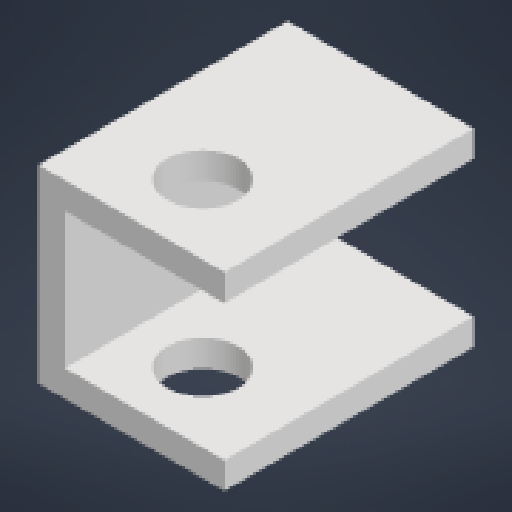
# Autodesk Inventor part: Part4
Saved by Autodesk Inventor 2026 (Build 300175000, 175)
## iProperties
Created: 2025-10-10
Part Number: Part4
Material: Generic
Document SubType Name: Modeling
Designer: kenny
Density: 1 g/cm^3
Appearance: Default
Author: kenny
Autodesk Inventor part; units mm, degrees
ref_plane "YZ Plane" through (0, 0, 0) normal (1, 0, 0) x (0, 1, 0)
ref_plane "XZ Plane" through (0, 0, 0) normal (0, 1, 0) x (-1, 0, 0)
ref_plane "XY Plane" through (0, 0, 0) normal (0, 0, 1) x (1, 0, 0)
sketch "Sketch1" plane through (0, 0, 0) normal (0, 0, 1) x (1, 0, 0)
  line L0 (-5.7, 0) -> (-5.7, -5.7)
  line L1 (-5.7, -5.7) -> (0, -5.7)
  line L2 (0, 5.7) -> (-5.7, 5.7)
  line L3 (-5.7, 5.7) -> (-5.7, 0)
  line L4 (0, 4.1) -> (-4.1, 4.1)
  line L5 (-4.1, 4.1) -> (-4.1, -4.1)
  line L6 (-4.1, -4.1) -> (0, -4.1)
  line L7 (3.9, -5.7) -> (0, -5.7)
  line L8 (3.9, 5.7) -> (0, 5.7)
  line L9 (3.9, 5.7) -> (5.5, 5.7)
  line L10 (3.9, -5.7) -> (5.5, -5.7)
  line L11 (5.5, 4.1) -> (0, 4.1)
  line L12 (5.5, -4.1) -> (0, -4.1)
  line L13 (0, 0) -> (4.1, 0)
  line L14 (4.1, 0) -> (5.7, 0)
  line L15 (5.7, 0) -> (5.7, 5.7)
  line L16 (5.7, 5.7) -> (5.5, 5.7)
  line L17 (5.5, 4.1) -> (5.7, 4.1)
  line L18 (5.7, 0) -> (5.7, -5.7)
  line L19 (5.7, -5.7) -> (5.5, -5.7)
  line L20 (5.5, -4.1) -> (5.7, -4.1)
  dimension "d22" = 4.1
  dimension "d23" = 1.6
  constraints: 42 end point, 8 perpendicular, 5 point on line, 3 horizontal, 2 collinear
  measures "d22" distance of L13.start L13.end
  measures "d23" distance of L13.end L14.end
extrude "Extrusion1" add sketch "Sketch1" against normal blind 15 contours L3 L2 L8 L9 L16 L15 L17 L11 L4 L5 L6 L12 L20 L18 L19 L10 L7 L1 L0
sketch "Sketch2" plane through (-5.7, 5.7, 0) normal (0, 1, 0) x (1, 0, 0)
  line L0 (5.7, 0) -> (5.7, 4.2)
  circle A0 centre (5.7, 4.2) radius 2.15
  dimension "d10" = 4.2
  dimension "d11" = 4.3
  constraints: 2 end point, 1 centre point, 1 coincident, 1 vertical
  measures "d10" distance of L0.start L0.end
  measures "d11" diameter of A0
extrude "Extrusion2" cut sketch "Sketch2" against normal blind 15
sketch "Sketch3" plane through (0, 0, 0) normal (0, 0, 1) x (1, 0, 0)
  point P0 (0, 0)
sketch "Sketch4" plane through (0, 0, 0) normal (0, 0, 1) x (1, 0, 0)
  point P0 (5.5, 5.7)
sketch "Sketch5" plane through (0, 0, 0) normal (0, 0, 1) x (1, 0, 0)
  line L0 (5.7, 4.1) -> (5.7, 0)
  line L1 (5.7, 0) -> (5.7, 24)
  line L2 (5.7, 0) -> (5.7, -24)
  line L3 (5.7, -25.6) -> (4.1, -25.6)
  line L4 (5.7, -5.7) -> (-5.7, -5.7) projected
  line L5 (4.1, -5.7) -> (4.1, -25.6)
  line L6 (5.7, 25.6) -> (4.1, 25.6)
  line L7 (4.1, 25.6) -> (4.1, 5.7)
  line L8 (5.7, 5.7) -> (-5.7, 5.7) projected
  line L9 (5.7, 25.6) -> (18.7, 25.6)
  line L10 (18.7, 25.6) -> (18.7, 24)
  line L11 (18.7, 24) -> (5.7, 24)
  line L12 (5.7, -25.6) -> (18.7, -25.6)
  line L13 (18.7, -25.6) -> (18.7, -24)
  line L14 (18.7, -24) -> (5.7, -24)
  line L15 (4.1, 5.7) -> (4.1, -5.7)
  line L16 (5.7, -4.1) -> (-4.1, -4.1) projected
  line L17 (4.1, 5.7) -> (5.7, 5.7)
  line L18 (4.1, 4.1) -> (5.7, 4.1)
  line L19 (4.1, -4.1) -> (5.7, -4.1)
  line L20 (4.1, -5.7) -> (5.7, -5.7)
  point P0 (0, 0)
  constraints: 36 end point, 10 point on line, 5 perpendicular, 3 collinear, 2 vertical, 1 parallel
extrude "Extrusion3" add sketch "Sketch5" against normal blind 15 contours L8 L7 L6 L9 L10 L11 L1 | L2 L14 L13 L12 L3 L5 L4
sketch "Sketch6" plane through (0, 0, 0) normal (0, 0, 1) x (1, 0, 0)
  line L0 (18.7, -25.6) -> (4.1, -25.6) projected
  line L1 (4.1, -25.6) -> (4.1, 4.1)
  line L2 (5.7, 4.1) -> (-4.1, 4.1) projected
  line L3 (5.7, -4.1) -> (5.7, -24) projected
  line L4 (5.7, 4.1) -> (5.7, -24)
  line L5 (4.1, -25.6) -> (18.7, -25.6)
  line L6 (18.7, -24) -> (18.7, -25.6) projected
  line L7 (18.7, -24) -> (5.7, -24) projected
  line L8 (18.7, -24) -> (5.7, -24)
  line L9 (5.7, 4.1) -> (5.7, 24) projected
  line L10 (5.7, 4.1) -> (5.7, 24)
  line L11 (5.7, 24) -> (18.7, 24)
  line L12 (18.7, 25.6) -> (4.1, 25.6) projected
  line L13 (18.7, 24) -> (18.7, 25.6) projected
  line L14 (18.7, 25.6) -> (18.7, 24)
  line L15 (18.7, 25.6) -> (4.1, 25.6)
  line L16 (4.1, 4.1) -> (4.1, 25.6)
  line L17 (4.1, 5.7) -> (-5.7, 5.7) projected
  point P0 (0, 0)
  constraints: 18 end point, 6 collinear, 2 perpendicular, 1 point on line, 1 vertical
extrude "Extrusion4" add sketch "Sketch6" along normal blind 18.6
sketch "Sketch7" plane through (5.7, 4.1, -15) normal (1, 0, 0) x (0, 0, -1)
  line L0 (0, -28.1) -> (-33.6, -28.1) projected
  line L1 (-33.6, -28.1) -> (-33.6, 19.9) projected
  line L2 (-33.6, -28.1) -> (-33.6, 19.9)
  line L3 (-33.6, 19.9) -> (-32, 19.9)
  line L4 (0, 19.9) -> (-33.6, 19.9) projected
  line L5 (-32, 19.9) -> (-32, -28.1)
  line L6 (-32, -28.1) -> (-33.6, -28.1)
  point P0 (-15, -4.1)
  dimension "d35" = 1.6
  constraints: 8 end point, 2 perpendicular, 1 collinear, 1 point on line
  measures "d35" distance of L1.end L3.end
extrude "Extrusion5" add sketch "Sketch7" along normal blind 13
sketch "Sketch8" plane through (5.7, -24, -15) normal (1, 0, 0) x (0, 0, -1)
  line L0 (0, 0) -> (0, -1.6) projected
  line L1 (-8.4022, 0) -> (-11.0502, 0)
  line L2 (-32, 0) -> (0, 0) projected
  line L3 (-11.0502, 0) -> (-10.0022, 0)
  line L4 (-10.0022, 0) -> (-10.0022, 18.3)
  line L5 (0, 18.3) -> (-15, 18.3) projected
  line L6 (0, 49.6) -> (-33.6, 49.6) projected
  line L7 (-8.4022, 49.6) -> (-10.0022, 49.6)
  line L8 (-15, 29.7) -> (0, 29.7) projected
  line L9 (-10.0022, 29.7) -> (-10.0022, 49.6)
  line L10 (-10.0022, 0) -> (-10.0022, 18.3)
  line L11 (-10.0022, 29.7) -> (-10.0022, 48)
  line L12 (-32, 48) -> (0, 48) projected
  line L13 (-10.0022, 0) -> (-8.4022, 0)
  line L14 (-8.4022, 0) -> (-8.4022, 18.3)
  line L15 (-8.4022, 29.7) -> (-8.4022, 48)
  line L16 (-10.0022, 18.3) -> (-8.4022, 18.3)
  line L17 (-10.0022, 29.7) -> (-8.4022, 29.7)
  line L18 (-10.0022, 48) -> (-8.4022, 48)
  line L19 (-10.0022, 0) -> (-8.4022, 0)
  point P0 (-15, 24)
  dimension "d38" = 1.6
  constraints: 28 end point, 14 point on line, 4 collinear, 3 perpendicular
  measures "d38" distance of L1.start L3.end
extrude "Extrusion6" add sketch "Sketch8" along normal blind 8
sketch "Sketch9" plane through (5.7, 24, -15) normal (0, -1, 0) x (1, 0, 0)
  line L0 (13, 0) -> (0, 0) projected
  line L1 (13, 0) -> (13, 1.6)
  line L2 (13, 32) -> (13, 0) projected
  line L3 (13, 1.6) -> (0, 1.6)
  line L4 (0, 0) -> (0, 8.4022) projected
  line L5 (0, 0) -> (0, 1.6)
  line L6 (-1.6, 0) -> (13, 0) projected
  line L7 (0, 0) -> (13, 0)
  point P0 (-5.7, 15)
  dimension "d41" = 1.6
  constraints: 8 end point, 2 perpendicular, 2 point on line, 1 horizontal
  measures "d41" distance of L0.start L1.end
extrude "Extrusion7" add sketch "Sketch9" along normal blind 48
sketch "Sketch10" plane through (18.7, -25.6, -15) normal (1, 0, 0) x (0, 0, -1)
  point P0 (-15, 25.6)
sketch "Sketch11" plane through (5.7, 24, 17) normal (0, -1, 0) x (1, 0, 0)
  line L0 (8, -23.5978) -> (8, -26.9978)
  line L1 (0, -30.4) -> (13, -30.4) projected
  circle A0 centre (8, -26.9978) radius 2.05
  point P0 (-5.7, -17)
  dimension "d44" = 3.4
  dimension "d45" = 4.1
  constraints: 2 end point, 1 centre point, 1 coincident, 1 perpendicular
  measures "d44" distance of L0.start L0.end
  measures "d45" diameter of A0
extrude "Extrusion8" cut sketch "Sketch11" along normal blind 59
extrude "Extrusion9" cut sketch "Sketch11" against normal blind 18
body "Solid1"
